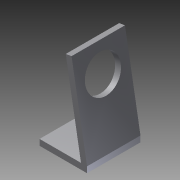
# Autodesk Inventor part: bunny throw piston bracket
Saved by Autodesk Inventor 2012 (Build 160160000, 160)
## iProperties
Created: 2013-10-11
Part Number: bunny throw piston bracket
Material: Default
Document SubType Name: Modeling
Designer: Bryce
Density: 1 g/cm^3
Author: Bryce
Autodesk Inventor part; units mm, degrees
ref_plane "YZ Plane" through (0, 0, 0) normal (1, 0, 0) x (0, 1, 0)
ref_plane "XZ Plane" through (0, 0, 0) normal (0, 1, 0) x (-1, 0, 0)
ref_plane "XY Plane" through (0, 0, 0) normal (0, 0, 1) x (1, 0, 0)
sketch "Sketch1" plane through (0, 0, 0) normal (0, 0, 1) x (1, 0, 0)
  line L0 (0, 0) -> (0, 3.175)
  line L1 (0, 0) -> (25.4, 0)
  line L2 (25.4, 0) -> (25.4, 3.175)
  line L3 (25.4, 3.175) -> (17.13, 50.0765)
  line L4 (17.13, 50.0765) -> (14.0032, 49.5251)
  line L5 (14.0032, 49.5251) -> (22.176, 3.175)
  line L6 (0, 3.175) -> (22.176, 3.175)
  dimension "d0" = 3.175
  dimension "d1" = 25.4
  dimension "d3" = 3.175
  dimension "d4" = 80
  dimension "d5" = 47.625
  constraints: 14 end point, 5 perpendicular, 1 parallel, 1 vertical
  measures "d0" distance of L0.start L0.end
  measures "d1" distance of L0.start L1.end
  measures "d3" distance of L3.end L4.end
  measures "d4" angle of L6 L5
  measures "d5" distance of L2.end L3.end
extrude "Extrusion1" add sketch "Sketch1" along normal blind 28.575
sketch "Sketch2" plane through (14.0032, 49.5251, 0) normal (-0.9848078, -0.1736482, 0) x (0, 0, 1)
  line L0 (28.575, -47.0652) -> (28.575, 0) projected
  line L1 (0, 0) -> (28.575, 0) projected
  circle A0 centre (14.2875, -14.2875) radius 9.525
  point P0 (0, -46.3411)
  dimension "d8" = 19.05
  dimension "d9" = 14.2875
  dimension "d10" = 14.2875
  constraints: 1 centre point
  measures "d8" diameter of A0
  measures "d9" distance from line of L0 A0.centre
  measures "d10" distance from line of L1 A0.centre
extrude "Extrusion2" cut sketch "Sketch2" against normal blind 28.575
equation "\"d3\" = d0"
equation "\"d10\" = d9"
body "Solid1"
